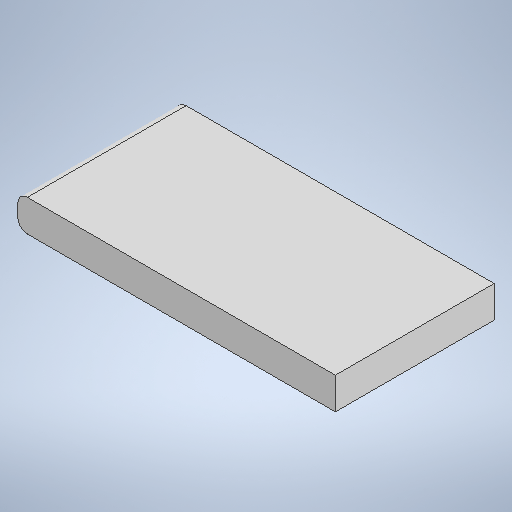
# Autodesk Inventor part: 13042025-02
Saved by Autodesk Inventor 2025.3 (Build 293356000, 356)
## iProperties
Created: 2026-04-13
Part Number: 13042025-02
Material: Generic
Document SubType Name: Modeling
Designer: Oski
Density: 1 g/cm^3
Appearance: Default
Author: Oski
Autodesk Inventor part; units mm, degrees
ref_plane "YZ Plane" through (0, 0, 0) normal (1, 0, 0) x (0, 1, 0)
ref_plane "XZ Plane" through (0, 0, 0) normal (0, 1, 0) x (-1, 0, 0)
ref_plane "XY Plane" through (0, 0, 0) normal (0, 0, 1) x (1, 0, 0)
sketch "Sketch1" plane through (0, 0, 0) normal (0, 0, 1) x (1, 0, 0)
  line L0 (-5, 5) -> (95, 5)
  line L1 (95, 5) -> (95, -5)
  line L2 (95, -5) -> (-5, -5)
  line L3 (-5, -5) -> (-5, 5)
  line L4 (0, 0) -> (0, 5) construction
  line L5 (0, 0) -> (0, -5) construction
  line L6 (0, 0) -> (-5, 0) construction
  dimension "d0" = 100
  dimension "d1" = 10
  constraints: 14 end point, 3 perpendicular, 3 point on line, 2 equal length, 2 parallel, 1 horizontal, 1 midpoint
  measures "d0" distance of L0.start L0.end
  measures "d1" distance of L2.end L0.start
extrude "Extrusion1" add sketch "Sketch1" along normal blind 50
fillet "Fillet1" radius 3 2 edges at (-5, -5, 25) (-5, 5, 25)
body "Solid1"
